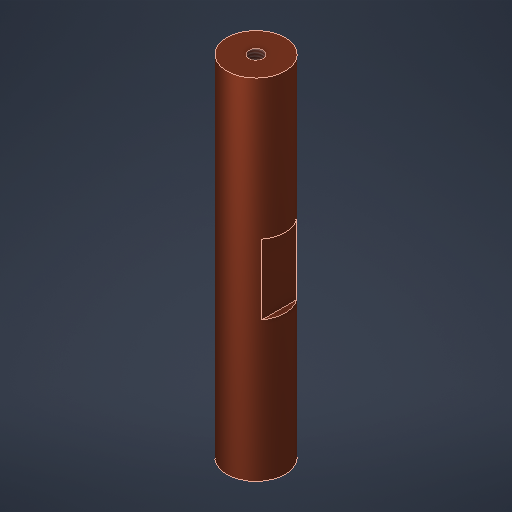
# Autodesk Inventor part: Post-2023-1
Saved by Autodesk Inventor 2026 (Build 300175050, 175E)
## iProperties
Created: 2018-11-20
Part Number: Post-2023-1
Material: Copper
Document SubType Name: Modeling
Designer: schanen
Density: 8.94 g/cm^3
Appearance: Copper - Satin
Mass: 40.8342 g
Surface Area: 22.7537 cm^2
Volume: 4.56758 cm^3
Author: schanen
Autodesk Inventor part; units mm, degrees
ref_plane "YZ Plane" through (0, 0, 0) normal (1, 0, 0) x (0, 1, 0)
ref_plane "XZ Plane" through (0, 0, 0) normal (0, 1, 0) x (-1, 0, 0)
ref_plane "XY Plane" through (0, 0, 0) normal (0, 0, 1) x (1, 0, 0)
sketch "Sketch1" plane through (0, 0, 0) normal (0, 1, 0) x (-1, 0, 0)
  circle A0 centre (0, 0) radius 5
  dimension "d0" = 10
  constraints: 1 centre point, 1 coincident
  measures "d0" diameter of A0
extrude "Extrusion1" add sketch "Sketch1" along normal blind 60
sketch "Sketch2" plane through (0, 60, 0) normal (0, 1, 0) x (1, 0, 0)
  point P0 (0, 0)
  point P1 (0, 0)
  constraints: 1 coincident
hole "Hole1" at (0, 60, 0) direction (0, -1, 0) diameter 2.459 depth 12 tip angle 118 thread size "M3x0.5" class "6H" standard "ANSI Metric M Profile"
sketch "Sketch3" plane through (0, 0, 0) normal (0, -1, 0) x (1, 0, 0)
  circle A0 centre (0, 0) radius 1.2295 projected
  constraints: 1 coincident
hole "Hole2" at (0, 0, 0) direction (0, 1, 0) diameter 2.459 depth 12 tip angle 118 thread size "M3x0.5" class "6H" standard "ANSI Metric M Profile"
sketch "Sketch4" plane through (0, 0, 0) normal (0, 0, 1) x (1, 0, 0)
  line L0 (-5, 0) -> (-5, 60) projected
  line L1 (5, 0) -> (5, 60) projected
  line L2 (-5, 0) -> (5, 0) projected
  line L3 (5, 60) -> (-5, 60) projected
  line L4 (-5, 24) -> (-4, 24)
  line L5 (-4, 24) -> (-4, 36)
  line L6 (-4, 36) -> (-5, 36)
  line L7 (5, 24) -> (4, 24)
  line L8 (4, 24) -> (4, 36)
  line L9 (4, 36) -> (5, 36)
  line L10 (-5, 36) -> (-15, 36)
  line L11 (-15, 36) -> (-15, 24)
  line L12 (-15, 24) -> (-5, 24)
  line L13 (5, 36) -> (15, 36)
  line L14 (15, 36) -> (15, 24)
  line L15 (15, 24) -> (5, 24)
  point P0 (0, 0)
  point P1 (-4.5, 24)
  dimension "d17" = 60
  dimension "d18" = 12
  dimension "d19" = 24
  dimension "d20" = 1
  dimension "d21" = 1
  dimension "d22" = 10
  dimension "d23" = 10
  constraints: 24 end point, 8 point on line, 7 perpendicular, 3 horizontal, 1 midpoint
  measures "d17" distance between parallel lines of L3 L2
  measures "d18" distance of L4.end L5.end
  measures "d19" distance from line of L2 point (-4.5, 24)
  measures "d20" distance between parallel lines of L0 L5
  measures "d21" distance between parallel lines of L1 L8
  measures "d22" distance of L6.end L10.end
  measures "d23" distance of L9.end L13.end
extrude "Extrusion2" cut sketch "Sketch4" along normal mid plane 10 contours L12 L11 L10 L0 | L0 L6 L5 L4 | L7 L8 L9 L1 | L1 L13 L14 L15
equation "\"d19\" = -0.5 * d18 + 0.5 * d17"
equation "\"d21\" = d20"
equation "\"d23\" = d22"
body "Solid1"
